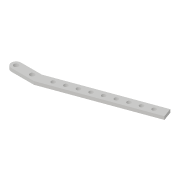
# Autodesk Inventor part: CollectorArm160
Saved by Autodesk Inventor 2018 (Build 220112000, 112)
## iProperties
Created: 2018-12-15
Part Number: CollectorArm160
Material: Generic
Document SubType Name: Modeling
Designer: ball
Density: 1 g/cm^3
Appearance: Default
Author: ball
Autodesk Inventor part; units mm, degrees
ref_plane "YZ Plane" through (0, 0, 0) normal (1, 0, 0) x (0, 1, 0)
ref_plane "XZ Plane" through (0, 0, 0) normal (0, 1, 0) x (-1, 0, 0)
ref_plane "XY Plane" through (0, 0, 0) normal (0, 0, 1) x (1, 0, 0)
sketch "Sketch1" plane through (0, 0, 0) normal (0, 1, 0) x (-1, 0, 0)
  line L0 (0, 0) -> (22.5402, 0)
  line L1 (22.5192, -9.525) -> (-0.0106, -9.525)
  line L2 (-0.0106, -9.525) -> (0, 0)
  arc A0 (22.5192, -9.525) -> (22.5402, 0) centre (22.4751, -4.7624) ccw
  line L3 (0, 0) -> (-95.0742, -34.6042)
  line L4 (0, 0) -> (101.1758, 0) construction
  line L5 (-95.0742, -34.6042) -> (-91.8164, -43.5547)
  line L6 (0, 0) -> (3.2577, -8.9506)
  line L7 (3.2577, -8.9506) -> (-91.8164, -43.5547)
  circle A1 centre (22.4751, -4.7624) radius 2.2479
  line L8 (22.4751, -4.7624) -> (6.4731, -4.7624) construction
  circle A2 centre (6.4731, -4.7624) radius 2.2479
  line L9 (1.6289, -4.4753) -> (-10.3052, -8.8189) construction
  circle A3 centre (-10.3052, -8.8189) radius 1.9685
  line L10 (1.6289, -4.4753) -> (-93.4453, -39.0795) construction
  circle A4 centre (-19.4945, -12.1636) radius 1.9685
  circle A5 centre (-28.6837, -15.5082) radius 1.9685
  circle A6 centre (-37.873, -18.8528) radius 1.9685
  circle A7 centre (-47.0622, -22.1974) radius 1.9685
  circle A8 centre (-56.2515, -25.542) radius 1.9685
  circle A9 centre (-65.4408, -28.8866) radius 1.9685
  circle A10 centre (-74.63, -32.2312) radius 1.9685
  circle A11 centre (-83.8193, -35.5759) radius 1.9685
  line L11 (22.4751, -4.7624) -> (6.4456, -4.7624) construction
  line L12 (6.4456, -4.7624) -> (6.4456, 11.2396) construction
  line L13 (6.4456, 11.2396) -> (22.4751, 11.2396) construction
  line L14 (22.4751, 11.2396) -> (22.4751, -4.7624) construction
  line L15 (14.4604, 11.2396) -> (14.4604, -4.7624) construction
  line L16 (22.4751, 3.2386) -> (6.4456, 3.2386) construction
  circle A12 centre (14.4604, 3.2386) radius 1.27 construction
  dimension "d0" = 22.5298
  dimension "d1" = 9.525
  dimension "d2" = 4.7628
  dimension "d4" = 160
  dimension "d7" = 9.525
  dimension "d8" = 9.525
  dimension "d9" = 4.4958
  dimension "d10" = 16.002
  dimension "d11" = 4.4958
  dimension "d12" = 12.7
  dimension "d13" = 3.937
  dimension "d14" = 4.7625
  dimension "d15" = 3.937
  dimension "d16" = 9.779
  dimension "d17" = 3.937
  dimension "d18" = 9.779
  dimension "d19" = 3.937
  dimension "d20" = 9.779
  dimension "d21" = 3.937
  dimension "d22" = 9.779
  dimension "d23" = 3.937
  dimension "d24" = 9.779
  dimension "d25" = 3.937
  dimension "d26" = 9.779
  dimension "d27" = 3.937
  dimension "d28" = 9.779
  dimension "d29" = 3.937
  dimension "d30" = 9.779
  dimension "d31" = 16.002
  dimension "d32" = 2.54
  dimension "d33" = 115.8874
  constraints: 32 end point, 13 centre point, 7 midpoint, 4 horizontal, 3 coincident, 3 parallel, 3 perpendicular, 2 point on circle, 1 equal length, 11 other
  measures "d0" distance of L1.start L1.end
  measures "d1" distance of L0.end L1.start
  measures "d2" radius of A0
  measures "d4" angle of L3 L4
  measures "d7" distance of L5.end L3.end
  measures "d8" distance of L0.start L6.end
  measures "d9" diameter of A1
  measures "d10" distance of L8.start L8.end
  measures "d11" diameter of A2
  measures "d12" distance of L9.start L9.end
  measures "d13" diameter of A3
  measures "d14" distance from line of L3 L9.end
  measures "d15" diameter of A4
  measures "d16" distance of A4.centre L9.end
  measures "d17" diameter of A5
  measures "d18" distance of A5.centre A4.centre
  measures "d19" diameter of A6
  measures "d20" distance of A6.centre A5.centre
  measures "d21" diameter of A7
  measures "d22" distance of A7.centre A6.centre
  measures "d23" diameter of A8
  measures "d24" distance of A8.centre A7.centre
  measures "d25" diameter of A9
  measures "d26" distance of A9.centre A8.centre
  measures "d27" diameter of A10
  measures "d28" distance of A10.centre A9.centre
  measures "d29" diameter of A11
  measures "d30" distance of A11.centre A10.centre
  measures "d31" distance of L11.end L12.end
  measures "d32" diameter of A12
  measures "d33" distance of L3.end A12.centre
extrude "Extrusion1" add sketch "Sketch1" along normal blind 3.175
body "Solid1"
